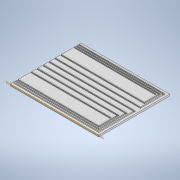
# Autodesk Inventor part: WIRE HOUSING
Saved by Autodesk Inventor 2020 (Build 240168000, 168)
## iProperties
Created: 2021-02-02
Part Number: WIRE HOUSING
Material: Generic
Document SubType Name: Modeling
Designer: apat475
Density: 1 g/cm^3
Appearance: Default
Author: apat475
Autodesk Inventor part; units mm, degrees
ref_plane "YZ Plane" through (0, 0, 0) normal (1, 0, 0) x (0, 1, 0)
ref_plane "XZ Plane" through (0, 0, 0) normal (0, 1, 0) x (-1, 0, 0)
ref_plane "XY Plane" through (0, 0, 0) normal (0, 0, 1) x (1, 0, 0)
sketch "Sketch1" plane through (0, 0, 0) normal (0, 1, 0) x (-1, 0, 0)
  line L0 (-135.9557, -16) -> (-525.9557, -16)
  line L1 (-525.9557, -16) -> (-525.9557, 150)
  line L2 (-135.9557, -11) -> (-520.9557, -11)
  line L3 (-520.9557, -11) -> (-520.9557, 145)
  line L4 (-510.9557, 16) -> (-510.9557, 135)
  line L5 (-515.9557, 11) -> (-515.9557, 140)
  line L6 (-500.9557, 43) -> (-500.9557, 125)
  line L7 (-505.9557, 38) -> (-505.9557, 130)
  line L8 (-495.9557, 70) -> (-495.9557, 65)
  line L9 (-535.9557, 160) -> (-135.9557, 160)
  line L10 (-135.9557, 160) -> (-135.9557, -160)
  line L11 (-135.9557, -160) -> (-535.9557, -160)
  line L12 (-535.9557, -160) -> (-535.9557, 160)
  line L13 (-525.9557, -150) -> (-525.9557, -38)
  line L14 (-520.9557, -145) -> (-520.9557, -43)
  line L15 (-510.9557, -135) -> (-510.9557, -70)
  line L16 (-515.9557, -140) -> (-515.9557, -65)
  line L17 (-505.9557, -130) -> (-505.9557, -125)
  line L18 (-525.9557, 150) -> (-135.9557, 150)
  line L19 (-520.9557, 145) -> (-135.9557, 145)
  line L20 (-515.9557, 140) -> (-135.9557, 140)
  line L21 (-505.9557, 130) -> (-135.9557, 130)
  line L22 (-500.9557, 125) -> (-135.9557, 125)
  line L23 (-510.9557, 135) -> (-135.9557, 135)
  line L24 (-135.9557, 70) -> (-495.9557, 70)
  line L25 (-135.9557, 65) -> (-495.9557, 65)
  line L26 (-135.9557, 43) -> (-500.9557, 43)
  line L27 (-135.9557, 38) -> (-505.9557, 38)
  line L28 (-135.9557, 16) -> (-510.9557, 16)
  line L29 (-135.9557, 11) -> (-515.9557, 11)
  line L30 (-525.9557, -38) -> (-135.9557, -38)
  line L31 (-520.9557, -43) -> (-135.9557, -43)
  line L32 (-515.9557, -65) -> (-135.9557, -65)
  line L33 (-510.9557, -70) -> (-135.9557, -70)
  line L34 (-135.9557, -125) -> (-505.9557, -125)
  line L35 (-135.9557, -130) -> (-505.9557, -130)
  line L36 (-135.9557, -135) -> (-510.9557, -135)
  line L37 (-135.9557, -140) -> (-515.9557, -140)
  line L38 (-135.9557, -145) -> (-520.9557, -145)
  line L39 (-135.9557, -150) -> (-525.9557, -150)
  dimension "d2" = 5
  dimension "d6" = 5
  dimension "d13" = 5
  dimension "d17" = 5
  dimension "d23" = 5
  dimension "d24" = 5
  dimension "d30" = 400
  dimension "d31" = 320
  dimension "d35" = 5
  dimension "d40" = 5
  dimension "d43" = 5
  dimension "d46" = 5
  dimension "d52" = 10
  dimension "d53" = 10
  constraints: 78 end point, 11 perpendicular, 8 horizontal, 6 parallel, 4 vertical, 27 other
  measures "d2" distance between parallel lines of L1 L3
  measures "d6" distance between parallel lines of L3 L5
  measures "d13" distance between parallel lines of L5 L4
  measures "d17" distance between parallel lines of L4 L7
  measures "d23" distance between parallel lines of L7 L6
  measures "d24" distance between parallel lines of L6 L8
  measures "d30" distance of L9.start L9.end
  measures "d31" distance of L11.end L9.start
  measures "d35" distance between parallel lines of L13 L14
  measures "d40" distance between parallel lines of L16 L15
  measures "d43" distance between parallel lines of L14 L16
  measures "d46" distance between parallel lines of L15 L17
  measures "d52" distance between parallel lines of L12 L13
  measures "d53" distance between parallel lines of L12 L1
extrude "Extrusion1" add sketch "Sketch1" against normal blind 5 contours L10 L30 L13 L39 L11 L12 L9 L18 L1 L0 | L2 L3 L19 L10 L20 L5 L29 | L10 L32 L16 L37 L38 L14 L31 | L28 L4 L23 L10 L21 L7 L27 | L10 L34 L17 L35 L36 L15 L33 | L26 L6 L22 L10 L24 L8 L25
ref_plane "Work Plane2" through (135.9557, 0, 160) normal (0, 0, 1) x (1, 0, 0)
sketch "Sketch3" plane through (135.9557, 0, 160) normal (0, 0, 1) x (1, 0, 0)
  line L0 (0, 0) -> (0, -5) projected
  line L1 (0, -5) -> (400, -5)
  line L2 (400, -5) -> (400, -8)
  line L3 (400, -8) -> (0, -8)
  line L4 (0, -8) -> (0, -5)
  point P0 (-135.9557, 0)
  dimension "d62" = 3
  constraints: 8 end point, 2 parallel, 1 horizontal, 1 perpendicular
  measures "d62" distance of L1.end L2.end
extrude "Extrusion3" add sketch "Sketch3" against normal blind 320
equation "\"d2\" = d25"
equation "\"d6\" = d26"
equation "\"d13\" = d25"
equation "\"d17\" = d26"
equation "\"d23\" = d25"
equation "\"d24\" = d26"
equation "\"d35\" = d47"
equation "\"d40\" = d47"
equation "\"d43\" = d49"
equation "\"d46\" = d49"
equation "\"d3\" = d25"
equation "\"d4\" = d25"
equation "\"d5\" = d26"
equation "\"d7\" = d25"
equation "\"d8\" = d25"
equation "\"d9\" = d25"
equation "\"d10\" = d26"
equation "\"d12\" = d28"
equation "\"d14\" = d25"
equation "\"d15\" = d28"
equation "\"d16\" = d26"
equation "\"d18\" = d25"
equation "\"d19\" = d25"
equation "\"d20\" = d28"
equation "\"d21\" = d25"
equation "\"d22\" = d25"
equation "\"d25\" = 5"
equation "\"d26\" = 5"
equation "\"d28\" = -1.2 * d25 + 0.2 * d29"
equation "\"d34\" = d47"
equation "\"d36\" = d47"
equation "\"d37\" = d48"
equation "\"d38\" = d47"
equation "\"d39\" = d49"
equation "\"d41\" = d47"
equation "\"d42\" = d48"
equation "\"d44\" = d47"
equation "\"d45\" = d49"
equation "\"d47\" = 5"
equation "\"d48\" = -1.2 * d47 + 0.2 * d50"
equation "\"d49\" = 5"
equation "\"d29\" = 140"
equation "\"d50\" = 140"
body "Solid1"
